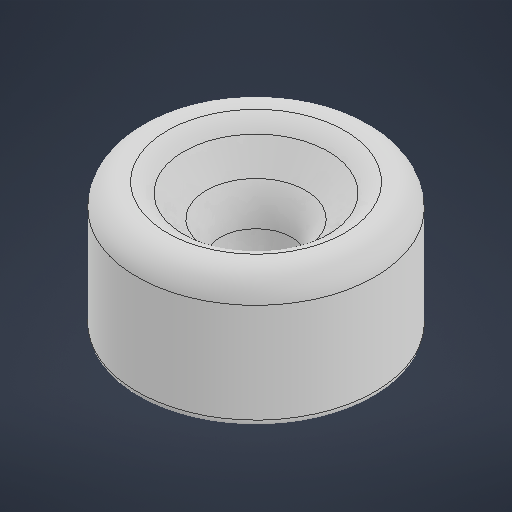
# Autodesk Inventor part: TransformerLug
Saved by Autodesk Inventor 2026.2 (Build 302298010, 298A)
## iProperties
Created: 2026-03-07
Part Number: TransformerLug
Material: Generic
Document SubType Name: Modeling
Designer: DanAr
Density: 1 g/cm^3
Appearance: Default
Author: DanAr
Autodesk Inventor part; units mm, degrees
ref_plane "YZ Plane" through (0, 0, 0) normal (1, 0, 0) x (0, 1, 0)
ref_plane "XZ Plane" through (0, 0, 0) normal (0, 1, 0) x (-1, 0, 0)
ref_plane "XY Plane" through (0, 0, 0) normal (0, 0, 1) x (1, 0, 0)
sketch "Sketch1" plane through (0, 0, 0) normal (0, 1, 0) x (-1, 0, 0)
  circle A0 centre (0, 0) radius 5
  circle A1 centre (0, 0) radius 1.5
  dimension "d0" = 10
  dimension "d1" = 3
  constraints: 2 centre point, 2 coincident
  measures "d0" diameter of A0
  measures "d1" diameter of A1
extrude "Extrusion1" add sketch "Sketch1" along normal blind 5.5
chamfer "Chamfer1" distance 2 angle 45 1 edges at (1.5, 5.5, 0)
fillet "Fillet1" radius 2 1 edges at (1.5, 3.5, 0)
fillet "Fillet2" radius 1.6 1 edges at (3.5, 5.5, 0)
fillet "Fillet3" radius 1 1 edges at (5, 5.5, 0)
fillet "Fillet4" radius 0.3 1 edges at (5, 0, 0)
fillet "Fillet5" radius 0.3 1 edges at (1.5, 0, 0)
body "Solid1"
